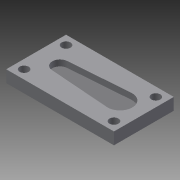
# Autodesk Inventor part: ServoHornHolder
Saved by Autodesk Inventor 2015 (Build 190159000, 159)
## iProperties
Created: 2014-09-29
Part Number: ServoHornHolder
Material: Generic
Document SubType Name: Modeling
Designer: Jaden
Density: 1 g/cm^3
Appearance: Default
Author: Jaden
Autodesk Inventor part; units mm, degrees
ref_plane "YZ Plane" through (0, 0, 0) normal (1, 0, 0) x (0, 1, 0)
ref_plane "XZ Plane" through (0, 0, 0) normal (0, 1, 0) x (-1, 0, 0)
ref_plane "XY Plane" through (0, 0, 0) normal (0, 0, 1) x (1, 0, 0)
sketch "Sketch1" plane through (0, 0, 0) normal (0, 0, 1) x (1, 0, 0)
  line L0 (-15.875, 28.575) -> (15.875, 28.575)
  line L1 (15.875, 28.575) -> (15.875, -28.575)
  line L2 (15.875, -28.575) -> (-15.875, -28.575)
  line L3 (-15.875, -28.575) -> (-15.875, 28.575)
  point P0 (0, 0)
  point P1 (15.875, 0)
  point P2 (0, 28.575)
  dimension "d0" = 31.75
  dimension "d1" = 57.15
  constraints: 8 end point, 2 midpoint, 2 parallel, 1 horizontal, 1 horizontal alignment, 1 perpendicular, 1 vertical alignment
  measures "d0" distance of L0.start L0.end
  measures "d1" distance of L0.end L1.end
extrude "Extrusion1" add sketch "Sketch1" along normal blind 6.35
sketch "Sketch2" plane through (0, 0, 6.35) normal (0, 0, 1) x (1, 0, 0)
  arc A0 (-6.4964, -15.4156) -> (6.4964, -15.4156) centre (0, -15.9071) ccw
  arc A1 (4.1031, 16.2175) -> (-4.1031, 16.2175) centre (0, 15.9071) ccw
  line L0 (4.1031, 16.2175) -> (6.4964, -15.4156)
  line L1 (-4.1031, 16.2175) -> (-6.4964, -15.4156)
  line L2 (-15.875, -28.575) -> (15.875, -28.575) projected
  line L3 (15.875, -28.575) -> (15.875, 28.575) projected
  dimension "d12" = 4.1148
  dimension "d13" = 6.515
  dimension "d18" = 4.327
  dimension "d23" = 15.875
  dimension "d24" = 31.8142
  dimension "d25" = 12.6679
  constraints: 4 end point, 4 point on circle, 4 tangent, 2 centre point
  measures "d12" radius of A1
  measures "d13" radius of A0
  measures "d18" angle of L0 L3
  measures "d23" distance from line of L3 A0.centre
  measures "d24" distance of A0.centre A1.centre
  measures "d25" distance from line of L2 A0.centre
extrude "Extrusion2" cut sketch "Sketch2" against normal blind 3.175
sketch "Sketch4" plane through (0, 0, 6.35) normal (0, 0, 1) x (1, 0, 0)
  line L0 (11.1125, 23.8125) -> (-11.1125, 23.8125)
  line L1 (-11.1125, 23.8125) -> (-11.1125, -23.8125)
  line L2 (-11.1125, -23.8125) -> (11.1125, -23.8125)
  line L3 (11.1125, -23.8125) -> (11.1125, 23.8125)
  line L4 (15.875, 28.575) -> (15.875, -28.575) projected
  line L5 (-15.875, -28.575) -> (15.875, -28.575) projected
  point P0 (0, 0)
  dimension "d42" = 4.7625
  dimension "d43" = 4.7625
  dimension "d44" = 47.625
  dimension "d45" = 22.225
  constraints: 8 end point, 2 parallel, 1 horizontal, 1 perpendicular
  measures "d42" distance between parallel lines of L4 L3
  measures "d43" distance between parallel lines of L5 L2
  measures "d44" distance of L0.end L1.end
  measures "d45" distance of L0.start L0.end
hole "Hole1" at (11.1125, 23.8125, 6.35) at (-11.1125, 23.8125, 6.35) at (-11.1125, -23.8125, 6.35) at (11.1125, -23.8125, 6.35) direction (0, 0, -1) diameter 4.7625 end through all
equation "\"d0\" = plate_width"
equation "\"d1\" = plate_height"
equation "\"d23\" = 0.5 * plate_width"
equation "\"d24\" = slot_centers"
equation "\"d25\" = -0.5 * slot_centers + 0.5 * plate_height"
equation "\"d42\" = hole_dist"
equation "\"d43\" = hole_dist"
equation "\"d44\" = plate_height - 2 * hole_dist"
equation "\"d45\" = plate_width - 2 * hole_dist"
equation "\"d46\" = hole_dia"
equation "\"plate_width\" = 31.75"
equation "\"plate_height\" = 57.15"
equation "\"slot_centers\" = 31.81417"
equation "\"hole_dia\" = 4.7625"
equation "\"hole_dist\" = 4.7625"
body "Solid1"
